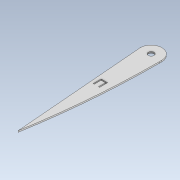
# Autodesk Inventor part: profil
Saved by Autodesk Inventor 2020 (Build 240168000, 168)
## iProperties
Created: 2020-09-11
Part Number: profil
Material: Generic
Document SubType Name: Modeling
Designer: Admin
Density: 1 g/cm^3
Appearance: Default
Author: Admin
Autodesk Inventor part; units mm, degrees
ref_plane "YZ Plane" through (0, 0, 0) normal (1, 0, 0) x (0, 1, 0)
ref_plane "XZ Plane" through (0, 0, 0) normal (0, 1, 0) x (-1, 0, 0)
ref_plane "XY Plane" through (0, 0, 0) normal (0, 0, 1) x (1, 0, 0)
sketch "Sketch1" plane through (0, 0, 0) normal (0, 1, 0) x (-1, 0, 0)
  line L0 (15, 0) -> (0, 0)
  line L1 (0, 0) -> (0, -200)
  line L2 (0, -200) -> (15, -200)
  line L3 (15, -200) -> (15, 0)
  dimension "d0" = 15
  dimension "d1" = 15
  dimension "d2" = 200
  constraints: 8 end point, 2 parallel, 1 horizontal, 1 perpendicular, 1 point on line
  measures "d0" distance of L0.start L0.end
  measures "d1" distance from line of point (0, 0) L3
  measures "d2" distance of L2.end L0.start
extrude "Extrusion1" add sketch "Sketch1" along normal blind 2
fillet "Fillet2" radius 15 1 edges at (0, 1, -200)
fillet "Fillet3" radius 1100 1 edges at (0, 1, 0)
mirror "Mirror1" about plane through (-15, 0, -200) normal (-1, 0, 0) of "Extrusion1"
fillet "Fillet5" radius 15 1 edges at (-30, 1, -200)
sketch "Sketch2" plane through (0, 0, 0) normal (0, -1, 0) x (1, 0, 0)
  line L0 (-15, 0) -> (-30, 0) projected
  line L1 (-30, 0) -> (-30, -185) projected
  line L2 (-15, 0) -> (-30, -185)
  line L3 (-30, -185) -> (-30, 0)
  arc A0 (0, -181.0387) -> (-15, 0) centre (-1100, -181.0387) ccw projected
  line L4 (-30, 0) -> (-15, 0)
  point P0 (0, 0)
  constraints: 6 end point, 1 collinear, 1 perpendicular
extrude "Extrusion2" cut sketch "Sketch2" against normal blind 2
sketch "Sketch3" plane through (0, 0, 0) normal (0, -1, 0) x (1, 0, 0)
  arc A0 (-30, -185) -> (0, -185) centre (-15, -185) ccw projected
  line L0 (0, -185) -> (-30, -185) construction
  circle A1 centre (-15, -185) radius 4
  line L1 (-10.5, -109) -> (-10.5, -120)
  line L2 (-10.5, -120) -> (-19.5, -120)
  line L3 (-19.5, -120) -> (-19.5, -109)
  line L4 (-19.5, -109) -> (-18, -109)
  line L5 (-18, -109) -> (-18, -118.4)
  line L6 (-18, -118.4) -> (-12, -118.4)
  line L7 (-12, -118.4) -> (-12, -109)
  line L8 (-12, -109) -> (-10.5, -109)
  point P0 (0, 0)
  dimension "d12" = 8
  dimension "d13" = 9
  dimension "d14" = 6
  dimension "d15" = 1.5
  dimension "d16" = 11
  dimension "d17" = 1.6
  dimension "d18" = 4.5
  dimension "d19" = 65
  constraints: 18 end point, 7 perpendicular, 1 centre point, 1 coincident, 1 horizontal, 1 point on line, 1 vertical
  measures "d12" diameter of A1
  measures "d13" distance of L1.end L2.end
  measures "d14" distance of L5.end L6.end
  measures "d15" distance between parallel lines of L7 L1
  measures "d16" distance of L1.start L1.end
  measures "d17" distance between parallel lines of L2 L6
  measures "d18" distance from line of A0.centre L1
  measures "d19" distance from line of A0.centre L2
extrude "Extrusion3" cut sketch "Sketch3" against normal blind 2
body "Solid1"
